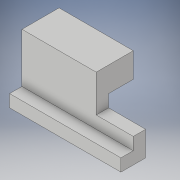
# Autodesk Inventor part: 4.1e P4
Saved by Autodesk Inventor 2017.1 (Build 211199000, 199)
## iProperties
Created: 2016-10-22
Part Number: 4.1e P4
Material: Generic
Document SubType Name: Modeling
Designer: rbibby53
Density: 1 g/cm^3
Appearance: Default
Author: rbibby53
Autodesk Inventor part; units mm, degrees
ref_plane "YZ Plane" through (0, 0, 0) normal (1, 0, 0) x (0, 1, 0)
ref_plane "XZ Plane" through (0, 0, 0) normal (0, 1, 0) x (-1, 0, 0)
ref_plane "XY Plane" through (0, 0, 0) normal (0, 0, 1) x (1, 0, 0)
sketch "Sketch1" plane through (0, 0, 0) normal (1, 0, 0) x (0, 1, 0)
  line L0 (10.991, 21.9414) -> (-14.409, 21.9414)
  line L1 (-14.409, 21.9414) -> (-14.409, -54.2586)
  line L2 (-14.409, -54.2586) -> (10.991, -54.2586)
  line L3 (10.991, -54.2586) -> (10.991, 21.9414)
  point P0 (0, 0)
  dimension "d0" = 25.4
  dimension "d1" = 76.2
  constraints: 8 end point, 2 parallel, 1 horizontal, 1 perpendicular
  measures "d0" distance of L2.end L1.end
  measures "d1" distance of L1.end L0.end
extrude "Extrusion1" add sketch "Sketch1" along normal blind 38.1
sketch "Sketch2" plane through (0, -14.409, -54.2586) normal (0, 0, -1) x (-1, 0, 0)
  line L0 (-38.1, 25.4) -> (-38.1, 0) projected
  line L1 (-38.1, 0) -> (-25.4, 0)
  line L2 (-25.4, 0) -> (-25.4, -12.7)
  line L3 (-25.4, -12.7) -> (-38.1, -12.7)
  line L4 (-38.1, -12.7) -> (-38.1, 0)
  point P0 (0, 14.409)
  dimension "d4" = 12.7
  dimension "d5" = 12.7
  constraints: 8 end point, 2 parallel, 1 horizontal, 1 perpendicular
  measures "d4" distance of L2.end L3.end
  measures "d5" distance of L1.end L2.end
extrude "Extrusion2" add sketch "Sketch2" against normal blind 76.2
sketch "Sketch3" plane through (0, -14.409, 21.9414) normal (0, 0, 1) x (1, 0, 0)
  line L0 (25.4, 0) -> (25.4, -12.7) projected
  line L1 (25.4, -12.7) -> (38.1, -12.7)
  line L2 (38.1, -12.7) -> (38.1, -38.1)
  line L3 (38.1, -38.1) -> (25.4, -38.1)
  line L4 (25.4, -38.1) -> (25.4, -12.7)
  point P0 (0, 14.409)
  dimension "d8" = 12.7
  dimension "d9" = 25.4
  constraints: 8 end point, 2 parallel, 1 horizontal, 1 perpendicular
  measures "d8" distance of L2.end L3.end
  measures "d9" distance of L1.end L2.end
extrude "Extrusion3" add sketch "Sketch3" against normal blind 114.3
sketch "Sketch4" plane through (38.1, 0, 0) normal (1, 0, 0) x (0, 0, -1)
  line L0 (-21.9414, -52.509) -> (92.3586, -52.509) projected
  line L1 (-21.9414, -52.509) -> (92.3586, -52.509)
  line L2 (92.3586, -52.509) -> (92.3586, -39.809)
  line L3 (92.3586, -39.809) -> (-21.9414, -39.809)
  line L4 (-21.9414, -39.809) -> (-21.9414, -52.509)
  point P0 (0, 0)
  dimension "d12" = 114.3
  dimension "d13" = 12.7
  constraints: 8 end point, 2 parallel, 1 horizontal, 1 perpendicular
  measures "d12" distance of L3.end L2.end
  measures "d13" distance of L2.end L1.end
extrude "Extrusion4" add sketch "Sketch4" along normal blind 12.7
body "Solid1"
